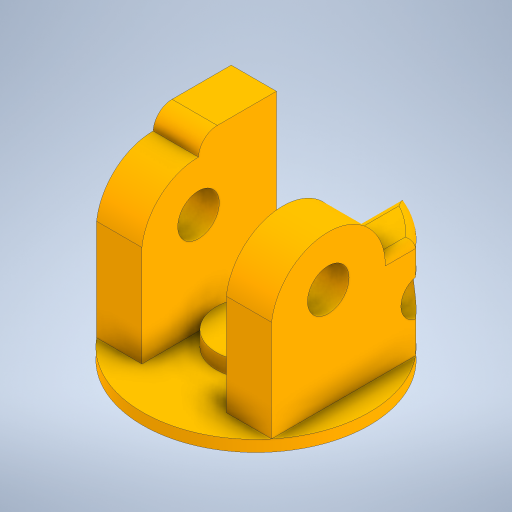
# Autodesk Inventor part: base2
Saved by Autodesk Inventor 2024 (Build 280153000, 153)
## iProperties
Created: 2024-04-28
Part Number: base2
Material: Generic
Document SubType Name: Modeling
Designer: samue
Density: 1 g/cm^3
Appearance: Default
Author: samue
## iProperties of the stored document base2_3DPrint.ipt
Created: 2024-04-28
Part Number: base2_3DPrint
Material: Generic
Document SubType Name: Modeling
Designer: samue
Density: 1 g/cm^3
Appearance: Default
Author: samue
Autodesk Inventor part; units mm, degrees
ref_plane "YZ Plane" through (0, 0, 0) normal (1, 0, 0) x (0, 1, 0)
ref_plane "XZ Plane" through (0, 0, 0) normal (0, 1, 0) x (-1, 0, 0)
ref_plane "XY Plane" through (0, 0, 0) normal (0, 0, 1) x (1, 0, 0)
sketch "Sketch1" plane through (0, 0, 0) normal (0, 1, 0) x (-1, 0, 0)
  circle A0 centre (0, 0) radius 30
  dimension "d0" = 60
  constraints: 1 centre point, 1 coincident
  measures "d0" diameter of A0
extrude "Extrusion1" add sketch "Sketch1" along normal blind 3
sketch "Sketch2" plane through (0, 3, 0) normal (0, 1, 0) x (1, 0, 0)
  circle A0 centre (0, 0) radius 5
  dimension "d3" = 10
  constraints: 1 centre point, 1 coincident
  measures "d3" diameter of A0
extrude "Extrusion2" cut sketch "Sketch2" against normal blind 4
sketch "Sketch4" plane through (0, 3, 0) normal (0, 1, 0) x (1, 0, 0)
  line L0 (-23.2158, -19.0158) -> (-11.2158, -19.0158)
  line L1 (-11.2158, -19.0158) -> (-11.2158, 10.9842)
  line L2 (-11.2158, 10.9842) -> (-23.2158, 10.9842)
  line L3 (-23.2158, 10.9842) -> (-23.2158, -19.0158)
  line L4 (-0.0289, -32.9889) -> (-0.0289, 43.4959) construction
  line L5 (23.1581, -19.0158) -> (11.1581, -19.0158)
  line L6 (11.1581, -19.0158) -> (11.1581, 10.9842)
  line L7 (11.1581, 10.9842) -> (23.1581, 10.9842)
  line L8 (23.1581, 10.9842) -> (23.1581, -19.0158)
  point P0 (0, -4.0158)
  point P1 (-23.2158, -4.0158)
  point P2 (23.2158, 0)
  dimension "d9" = 12
  dimension "d10" = 30
  constraints: 16 end point, 4 symmetric about line, 2 parallel, 1 horizontal, 1 horizontal alignment, 1 midpoint, 1 perpendicular, 1 vertical, 3 other
  measures "d9" distance of L2.end L1.end
  measures "d10" distance of L1.end L0.end
extrude "Extrusion4" add sketch "Sketch4" along normal blind 40
sketch "Sketch5" plane through (23.1581, 3, 19.0158) normal (1, 0, 0) x (0, 0, -1)
  line L0 (30, 0) -> (30, 40) projected
  line L1 (0, 0) -> (0, 40) projected
  arc A0 (30, 26.6004) -> (0, 26.7351) centre (14.9918, 24.8495) ccw
  line L2 (0, 26.7351) -> (0, 40)
  line L3 (30, 40) -> (0, 40) projected
  line L4 (30, 40) -> (30, 26.6004)
  point P0 (19.0158, -3)
  constraints: 4 end point, 2 point on circle, 2 point on line, 1 centre point, 1 collinear, 1 perpendicular
extrude "Extrusion5" cut sketch "Sketch5" against normal blind 74.5
sketch "Sketch6" plane through (23.1581, 3, 19.0158) normal (1, 0, 0) x (0, 0, -1)
  circle A0 centre (15, 26.7283) radius 5.5
  point P0 (19.0158, -3)
  dimension "d15" = 11
  constraints: 1 centre point
  measures "d15" diameter of A0
extrude "Extrusion6" cut sketch "Sketch6" against normal blind 74.5
sketch "Sketch7" plane through (23.1581, 3, 19.0158) normal (1, 0, 0) x (0, 0, -1)
  line L0 (30, 0) -> (30, 26.6004) projected
  line L1 (30, 26.6004) -> (49.0158, 26.6004)
  line L2 (49.0158, 0) -> (-10.9842, 0) projected
  line L3 (49.0158, 26.6004) -> (49.0158, 0)
  point P0 (19.0158, -3)
  point P1 (0, 0)
  point P2 (0.0152, 0)
  constraints: 4 end point, 1 horizontal, 1 vertical
extrude "Extrusion7" add sketch "Sketch7" against normal blind 12
sketch "Sketch8" plane through (23.1581, 3, 19.0158) normal (1, 0, 0) x (0, 0, -1)
  circle A0 centre (39.1574, 13.257) radius 4.9
  point P0 (19.0158, -3)
  dimension "d20" = 9.8
  constraints: 1 centre point
  measures "d20" diameter of A0
extrude "Extrusion8" cut sketch "Sketch8" against normal blind 12
sketch "Sketch9" plane through (23.1581, 3, -30) normal (0, -1, 0) x (1, 0, 0)
  line L0 (-12, 0) -> (-12, 2.1522) projected
  arc A0 (-12, 2.1522) -> (0, 10.929) centre (-23.1581, 30) ccw projected
  arc A1 (-12, 2.1522) -> (0, 10.929) centre (-23.1408, 29.9763) ccw
  line L1 (0, 10.929) -> (0, 0) projected
  line L2 (0, 10.929) -> (0, 0)
  line L3 (0, 0) -> (-12, 0)
  constraints: 4 end point, 2 point on circle, 1 centre point, 1 collinear, 1 perpendicular
extrude "Extrusion9" cut sketch "Sketch9" against normal blind 33.25
fillet "Fillet1" radius 2 3 edges at (23.1581, 29.6004, -15.0276) (17.7109, 29.6004, -24.2152) (11.1581, 29.6004, -19.416)
sketch "Sketch10" plane through (-11.2158, 3, -10.9842) normal (0, 0, -1) x (-1, 0, 0)
  line L0 (0, 0) -> (0, 26.7351) projected
  line L1 (12, 0) -> (12, 26.7351) projected
  line L2 (0, 26.7351) -> (12, 26.7351)
  line L3 (12, 26.7351) -> (12, 0)
  line L4 (12, 0) -> (0, 0)
  line L5 (0, 0) -> (0, 26.7351)
  point P0 (-11.2158, -3)
  constraints: 8 end point, 2 parallel, 1 horizontal, 1 perpendicular
extrude "Extrusion10" add sketch "Sketch10" along normal blind 5.656
sketch "Sketch11" plane through (-23.2158, 29.7351, -10.9842) normal (0, 1, 0) x (1, 0, 0)
  line L0 (12, -30) -> (12, 0) projected
  line L1 (0, -29.9848) -> (0, 5.656) projected
  line L2 (12, 0) -> (0, 0)
  line L3 (0, 0) -> (0, 5.656)
  line L4 (0, 5.656) -> (12, 5.656)
  line L5 (12, 5.656) -> (12, 0)
  point P0 (23.2158, -10.9842)
  point P1 (0, 0)
  constraints: 8 end point, 2 parallel, 1 horizontal, 1 perpendicular
extrude "Extrusion11" add sketch "Sketch11" along normal blind 18
sketch "Sketch12" plane through (-23.2158, 3, 19.0158) normal (-1, 0, 0) x (0, 0, 1)
  line L0 (-30, 44.7351) -> (-30, 26.6004) projected
  line L1 (-30, 44.7351) -> (-14.9918, 44.7351)
  line L2 (-14.9918, 44.7351) -> (-14.9918, 39.9594)
  arc A0 (0, 26.7351) -> (-30.0997, 24.6004) centre (-14.9918, 24.8495) ccw projected
  point P0 (-19.0158, -3)
  constraints: 4 end point, 1 horizontal, 1 perpendicular, 1 point on circle
extrude "Extrusion12" add sketch "Sketch12" against normal blind 12
fillet "Fillet2" radius 5 1 edges at (-17.2158, 47.7351, 4.024)
sketch "Sketch13" plane through (-11.2158, 3, -16.6402) normal (0, 0, -1) x (-1, 0, 0)
  circle A0 centre (6.3211, 10.551) radius 1
  circle A1 centre (6.3211, 41.2302) radius 1
  point P0 (-11.2158, -3)
  dimension "d33" = 2
  dimension "d34" = 2
  constraints: 2 centre point
  measures "d33" diameter of A0
  measures "d34" diameter of A1
extrude "Extrusion13" cut sketch "Sketch13" against normal blind 14
sketch "Sketch15" plane through (0, 3, 0) normal (0, 1, 0) x (1, 0, 0)
  circle A0 centre (0, 0) radius 5 projected
  circle A1 centre (0, 0) radius 10.5
  circle A2 centre (0, 0) radius 5
  dimension "d39" = 21
  constraints: 2 centre point, 2 coincident, 1 concentric
  measures "d39" diameter of A1
extrude "Extrusion15" add sketch "Sketch15" along normal blind 4
body "Solid1"
